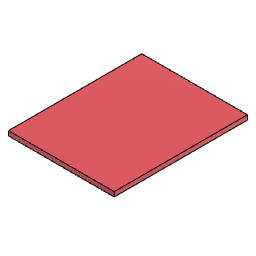
corte cajón 2 v13 (Autodesk Fusion 360 archive; units mm, degrees)
design "cajon_bottom"
Autodesk Fusion 360 part; units mm, degrees
sketch "Boceto1" plane through (0, 0, -56) normal (0, 0, -1) x (1, 0, 0)
  line L0 (-169, 102) -> (-31, 102)
  line L1 (-31, 102) -> (-31, 108)
  line L2 (-31, 108) -> (-169, 108)
  line L3 (-169, 108) -> (-169, 102)
  line L4 (-169, 108) -> (-31, 108)
  line L5 (-31, 108) -> (-31, -66)
  line L6 (-31, -66) -> (-169, -66)
  line L7 (-169, -66) -> (-169, 108)
  line L8 (-169, 102) -> (-169, -60)
  line L9 (-169, -66) -> (-31, -66)
  line L10 (-31, -60) -> (-31, 102)
  constraint horizontal L4
  constraint vertical L5
  constraint horizontal L6
  constraint vertical L7
  constraint collinear L2 L4
  constraint collinear L7 L8
  constraint collinear L6 L9
  constraint collinear L5 L10
sketch "Boceto2" plane through (0, 0, -62) normal (0, 0, -1) x (1, 0, 0)
  line L0 (-169, -66) -> (-31, -66)
  line L1 (-31, -66) -> (-31, 108)
  line L2 (-31, 108) -> (-169, 108)
  line L3 (-169, 108) -> (-169, -66)
  line L4 (-163, 102) -> (-37, 102)
  line L5 (-37, 102) -> (-37, -60)
  line L6 (-37, -60) -> (-163, -60)
  line L7 (-163, -60) -> (-163, 102)
  line L8 (-163, -60) -> (-163, 102)
  line L9 (-37, 102) -> (-37, -60)
  line L10 (-175, 102) -> (-25, 102)
  line L11 (-25, -60) -> (-175, -60)
  constraint horizontal L4
  constraint vertical L5
  constraint horizontal L6
  constraint vertical L7
  constraint collinear L7 L8
  constraint collinear L5 L9
  constraint collinear L4 L10
  constraint collinear L6 L11
extrude "Extruir1" add sketch "Boceto1" along normal blind 6
extrude "Extruir2" add sketch "Boceto2" along normal blind 6 contours L4 L5 L6 L7 L8 L9 L10 L11
